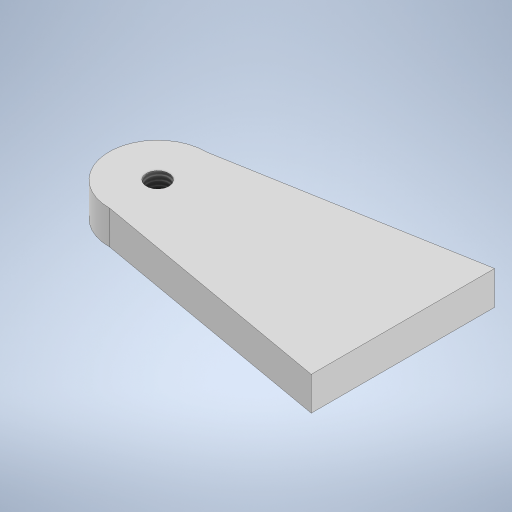
# Autodesk Inventor part: wea abajo movil
Saved by Autodesk Inventor 2023 (Build 270158000, 158)
## iProperties
Created: 2022-10-23
Part Number: wea abajo movil
Material: Generic
Document SubType Name: Modeling
Designer: User
Density: 1 g/cm^3
Appearance: Default
Author: User
Autodesk Inventor part; units mm, degrees
ref_plane "YZ Plane" through (0, 0, 0) normal (1, 0, 0) x (0, 1, 0)
ref_plane "XZ Plane" through (0, 0, 0) normal (0, 1, 0) x (-1, 0, 0)
ref_plane "XY Plane" through (0, 0, 0) normal (0, 0, 1) x (1, 0, 0)
sketch "Sketch1" plane through (0, 0, 0) normal (0, 1, 0) x (-1, 0, 0)
  line L0 (0, 0) -> (0, -30)
  line L1 (0, 0) -> (39.9996, -7.053)
  line L2 (0, -30) -> (39.9998, -22.947)
  arc A0 (39.9998, -22.947) -> (39.9996, -7.053) centre (40.1288, -15) ccw
  dimension "d0" = 30
  dimension "d1" = 80
  dimension "d4" = 80
  dimension "d7" = 15.896
  dimension "d9" = 40.1288
  dimension "d10" = 7.8038
  constraints: 6 end point, 2 point on circle, 1 centre point, 1 coincident, 1 vertical
  measures "d0" distance of L0.start L0.end
  measures "d1" angle of L1 L0
  measures "d4" angle of L0 L2
  measures "d7" diameter of A0
  measures "d9" distance from line of A0.centre L0
  measures "d10" distance from line of A0.centre L2
extrude "Extrusion1" add sketch "Sketch1" along normal blind 5.5
hole "Hole1" at (-40.1288, 0, -15) direction (0, 1, 0) diameter 3.6881 depth 13 tip angle 118 thread size "M4.5x0.75" class "6H" standard "ISO Metric profile"
body "Solid1"
